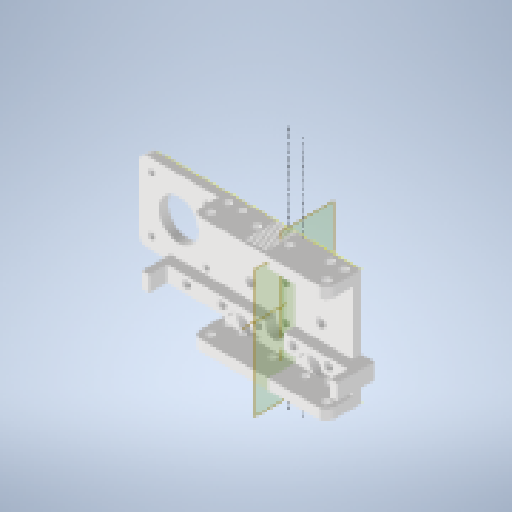
# Autodesk Inventor part: Frontside
Saved by Autodesk Inventor 2023 (Build 270158000, 158)
## iProperties
Created: 2023-08-31
Part Number: Frontside
Material: Generic
Document SubType Name: Modeling
Designer: Felix
Density: 1 g/cm^3
Appearance: Default
Author: Felix
Autodesk Inventor part; units mm, degrees
ref_plane "YZ Plane" through (0, 0, 0) normal (1, 0, 0) x (0, 1, 0)
ref_plane "XZ Plane" through (0, 0, 0) normal (0, 1, 0) x (-1, 0, 0)
ref_plane "XY Plane" through (0, 0, 0) normal (0, 0, 1) x (1, 0, 0)
ref_plane "Work Plane1" through (-29.75, -29.75, 0) normal (-1, 0, 0) x (0, 0, 1)
sketch "Sketch2" plane through (-29.75, -29.75, 0) normal (-1, 0, 0) x (0, 0, 1)
  line L0 (0, 32.5371) -> (-3, 32.5371) construction
  line L1 (0, -32.9629) -> (-3, -32.9629) construction
  line L2 (0, 32.5371) -> (5, 32.5371)
  line L3 (5, 32.5371) -> (5, -32.9629)
  line L4 (5, -32.9629) -> (0, -32.9629)
  line L5 (0, -32.9629) -> (0, 32.5371)
  line L6 (5, 32.5371) -> (20, 32.5371)
  line L7 (20, 32.5371) -> (20, 26.5371)
  line L8 (20, 26.5371) -> (5, 26.5371)
  line L9 (5, 26.5371) -> (5, 32.5371)
  line L10 (5, -32.9629) -> (20, -32.9629)
  line L11 (20, -32.9629) -> (20, -26.9629)
  line L12 (20, -26.9629) -> (5, -26.9629)
  line L13 (5, -26.9629) -> (5, -32.9629)
  point P0 (0, 29.75)
  point P1 (20, 29.5371)
  point P2 (5, 26.5371)
  dimension "d0" = 5
  dimension "d1" = 6
  dimension "d2" = 20
  dimension "d3" = 6
  dimension "d4" = 20
  constraints: 24 end point, 6 parallel, 3 horizontal, 3 perpendicular, 1 midpoint, 1 point on line
  measures "d0" distance of L3.end L4.end
  measures "d1" distance between parallel lines of L6 L8
  measures "d2" distance from line of point (20, 29.537) L5
  measures "d3" distance of L10.end L11.end
  measures "d4" distance between parallel lines of L5 L11
extrude "Extrusion1" add sketch "Sketch2" along normal mid plane 75.5
sketch "Sketch3" plane through (-67.5, -3.2129, 5) normal (0, 0, 1) x (1, 0, 0)
  circle A0 centre (17.6, -46.75) radius 2.5 construction
  circle A1 centre (57.6, -46.75) radius 3.6 construction
  circle A2 centre (17.6, -6.75) radius 2.5 construction
  circle A3 centre (57.6, -6.75) radius 3.6 construction
  point P0 (67.5, 3.2129)
hole "Hole1" at (-49.9, -49.9629, 5) at (-49.9, -9.9629, 5) at (-9.9, -9.9629, 5) at (-9.9, -49.9629, 5) direction (0, 0, -1) diameter 15 end through all
sketch "Sketch4" plane through (-67.5, -3.2129, 5) normal (0, 0, 1) x (1, 0, 0)
  circle A0 centre (57.6, -26.75) radius 3.6 construction
  circle A1 centre (17.9, -26.75) radius 2.55 construction
  point P0 (67.5, 3.2129)
hole "Hole2" at (-49.6, -29.9629, 5) at (-9.9, -29.9629, 5) direction (0, 0, -1) diameter 5.5 end through all clearance for "Countersunk Flat Head Screw DIN EN ISO 2009" size "M5" standard "DIN"
hole "Hole3" at (-29.75, -39.9629, 5) at (-29.75, -19.9629, 5) direction (0, 0, -1) diameter 4.5 end through all clearance for "Slotted Cheese Head Screw DIN 84" size "M4" standard "DIN"
sketch "Sketch6" plane through (-67.5, -3.2129, 5) normal (0, 0, 1) x (1, 0, 0)
  line L0 (0, 6) -> (0, -59.5) construction
  line L1 (75.5, -59.5) -> (75.5, 6) construction
  line L2 (0, -53.5) -> (0, 0) construction
  line L3 (-27.25, -44.5) -> (82.75, -44.5)
  line L4 (82.75, -44.5) -> (82.75, -35.5)
  line L5 (82.75, -35.5) -> (-27.25, -35.5)
  line L6 (-27.25, -35.5) -> (-27.25, -44.5)
  circle A0 centre (17.9, -26.75) radius 2.75 construction
  circle A1 centre (57.6, -26.75) radius 2.75 construction
  circle A2 centre (17.9, -26.75) radius 6.5
  circle A3 centre (57.6, -26.75) radius 6.5
  line L7 (75.5, -53.5) -> (0, -53.5) projected
  arc A4 (20.8692, -53.5) -> (14.3308, -53.5) centre (17.6, -46.75) ccw projected
  arc A5 (60.8692, -53.5) -> (54.3308, -53.5) centre (57.6, -46.75) ccw projected
  line L8 (-27.25, -40) -> (82.75, -40) construction
  line L9 (0, -26.75) -> (75.5, -26.75) construction
  circle A6 centre (37.75, -36.75) radius 2.25 projected
  circle A7 centre (37.75, -36.75) radius 2.25 projected
  circle A8 centre (37.75, -36.75) radius 5.5
  point P0 (67.5, 3.2129)
  point P1 (67.75, -40)
  point P2 (47.75, -40)
  point P3 (27.75, -40)
  point P4 (7.75, -40)
  point P5 (-12.25, -40)
  point P6 (52.8231, -32.1581)
  point P7 (62.2904, -32.25)
  point P8 (52.9096, -32.25)
  point P9 (62.3769, -32.1581)
  point P10 (13.1231, -32.1581)
  point P11 (22.5904, -32.25)
  point P12 (13.2096, -32.25)
  point P13 (22.6769, -32.1581)
  point P14 (37.75, -26.75)
  point P15 (10.4455, -44.5)
  point P16 (24.7545, -44.5)
  point P17 (50.4455, -44.5)
  point P18 (64.7545, -44.5)
  point P19 (43.1061, -35.5)
  point P20 (32.3939, -35.5)
  point P21 (35.8792, -35.5)
  point P22 (39.6208, -35.5)
  dimension "d28" = 20
  dimension "d29" = 20
  dimension "d30" = 20
  dimension "d31" = 20
  dimension "d33" = 9
  dimension "d34" = 110
  dimension "d36" = 15
  dimension "d38" = 13
  dimension "d39" = 13
  dimension "d56" = 15
  dimension "d57" = 9
  dimension "d58" = 10
  dimension "d59" = 11
  constraints: 12 end point, 6 midpoint, 4 point on line, 3 centre point, 3 coincident, 2 horizontal, 2 parallel, 1 perpendicular
  measures "d28" distance of point (-12.25, -40) point (7.75, -40)
  measures "d29" distance of point (7.75, -40) point (27.75, -40)
  measures "d30" distance of point (27.75, -40) point (47.75, -40)
  measures "d31" distance of point (47.75, -40) point (67.75, -40)
  measures "d33" distance between parallel lines of L5 L3
  measures "d34" distance between parallel lines of L6 L4
  measures "d36" distance from line of point (67.75, -40) L4
  measures "d38" diameter of A2
  measures "d39" diameter of A3
  measures "d56" distance from line of L6 point (-12.25, -40)
  measures "d57" distance between parallel lines of L7 L3
  measures "d58" horizontal distance of point (27.75, -40) point (37.75, -26.75)
  measures "d59" diameter of A8
extrude "Extrusion2" add sketch "Sketch6" along normal blind 6 and the other way blind 5 contours L6 L5 A8 L4 L3 A5 A4
sketch "Sketch7" plane through (-67.5, -3.2129, 11) normal (0, 0, 1) x (1, 0, 0)
  point P0 (67.5, 3.2129)
  point P1 (-12.25, -40)
  point P2 (7.75, -40)
  point P3 (27.75, -40)
  point P4 (47.75, -40)
  point P5 (67.75, -40)
hole "Hole4" at (-79.75, -43.2129, 11) at (-59.75, -43.2129, 11) at (-39.75, -43.2129, 11) at (-19.75, -43.2129, 11) at (0.25, -43.2129, 11) direction (0, 0, -1) diameter 4.3 end through all countersink diameter 5 countersink angle 90
sketch "Sketch8" plane through (-67.5, -3.2129, 11) normal (0, 0, 1) x (1, 0, 0)
  line L0 (-27.25, -35.5) -> (-27.25, -44.5) projected
  line L1 (82.75, -44.5) -> (82.75, -35.5) projected
  line L2 (82.75, -35.5) -> (-27.25, -35.5) construction
  line L3 (-27.25, -44.5) -> (82.75, -44.5) construction
  line L4 (-27.25, -35.5) -> (-23.25, -35.5)
  line L5 (-23.25, -35.5) -> (-23.25, -44.5)
  line L6 (-23.25, -44.5) -> (-27.25, -44.5)
  line L7 (-27.25, -44.5) -> (-27.25, -35.5)
  line L8 (82.75, -35.5) -> (-27.25, -35.5) construction
  line L9 (82.75, -44.5) -> (78.75, -44.5)
  line L10 (78.75, -44.5) -> (78.75, -35.5)
  line L11 (78.75, -35.5) -> (82.75, -35.5)
  line L12 (82.75, -35.5) -> (82.75, -44.5)
  point P0 (67.5, 3.2129)
  point P1 (13.2096, -23.25)
  point P2 (13.2096, -32.25)
  point P3 (62.2904, -23.25)
  dimension "d51" = 4
  dimension "d52" = 4
  constraints: 16 end point, 4 parallel, 2 horizontal, 2 perpendicular, 5 other
  measures "d51" distance of L5.end L6.end
  measures "d52" distance of L10.end L11.end
extrude "Extrusion3" add sketch "Sketch8" along normal blind 11
sketch "Sketch9" plane through (8, -62.7129, 0) normal (0, 0, -1) x (-1, 0, 0)
  line L0 (113.5, 58.5) -> (82.5, 58.5) construction
  line L1 (82.5, 58.5) -> (82.5, 27.5) construction
  line L2 (82.5, 27.5) -> (113.5, 27.5) construction
  line L3 (113.5, 27.5) -> (113.5, 58.5) construction
  line L4 (113.5, 58.5) -> (82.5, 27.5) construction
  line L5 (82.5, 58.5) -> (113.5, 27.5) construction
  line L6 (75.5, 65.5) -> (75.5, 24) construction
  line L7 (102.75, 24) -> (75.5, 24) construction
  line L8 (120.5, 20.5) -> (75.5, 20.5)
  line L9 (75.5, 20.5) -> (75.5, 65.5)
  line L10 (75.5, 65.5) -> (120.5, 65.5)
  line L11 (120.5, 65.5) -> (120.5, 20.5)
  line L12 (120.5, 20.5) -> (75.5, 65.5) construction
  line L13 (75.5, 20.5) -> (120.5, 65.5) construction
  circle A0 centre (98, 43) radius 11.25
  point P0 (8, 62.7129)
  dimension "d60" = 31
  dimension "d61" = 31
  dimension "d62" = 45
  dimension "d63" = 45
  dimension "d64" = 22.5
  constraints: 24 end point, 4 midpoint, 4 parallel, 2 horizontal, 2 perpendicular, 1 centre point, 1 coincident
  measures "d60" distance of L2.end L1.end
  measures "d61" distance of L1.end L0.end
  measures "d62" distance of L6.start L10.end
  measures "d63" distance of L6.start L8.end
  measures "d64" diameter of A0
extrude "Extrusion4" add sketch "Sketch9" against normal up to surface (5 mm away)
sketch "Sketch10" plane through (-67.5, -3.2129, 5) normal (0, 0, 1) x (1, 0, 0)
  point P0 (67.5, 3.2129)
  point P1 (-38, -1)
  point P2 (-38, -32)
  point P3 (-7, -32)
  point P4 (-7, -1)
hole "Hole5" at (-105.5, -35.2129, 5) at (-74.5, -35.2129, 5) at (-74.5, -4.2129, 5) at (-105.5, -4.2129, 5) direction (0, 0, -1) diameter 3.6 depth 8 clearance for "Countersunk Flat Head Screw DIN EN ISO 2009" size "M3" standard "DIN"
fillet "Fillet1" radius 5 8 edges at (-67.5, -52.2129, 5) (-67.5, -0.2129, 20) (-67.5, -59.7129, 20) (8, -59.7129, 20) (8, -0.2129, 20) (-94.75, -42.2129, 2.5) (-112.5, -42.2129, 2.5) (-112.5, 2.7871, 2.5)
ref_plane "Work Plane2" through (-24.7, -35.7634, 20.0758) normal (-1, 0, 0) x (0, 0, 1)
sketch "Sketch11" plane through (-24.7, -35.7634, 20.0758) normal (-1, 0, 0) x (0, 0, 1)
  line L0 (-20.0758, -26.9495) -> (-5.0758, -26.9495) construction
  line L1 (-20.0758, -27.1495) -> (-20.0758, -26.9495) construction
  line L2 (-5.0758, -26.9495) -> (-20.0758, -26.9495) construction
  line L3 (-19.0758, -27.1495) -> (-19.0758, -26.9495) construction
  arc A0 (-20.0758, -27.1495) -> (-19.0758, -27.1495) centre (-19.5758, -27.1495) ccw construction
  arc A1 (-18.0758, -27.1495) -> (-17.0758, -27.1495) centre (-17.5758, -27.1495) ccw construction
  line L4 (-18.0758, -27.1495) -> (-18.0758, -26.9495) construction
  line L5 (-17.0758, -27.1495) -> (-17.0758, -26.9495) construction
  arc A2 (-16.0758, -27.1495) -> (-15.0758, -27.1495) centre (-15.5758, -27.1495) ccw construction
  line L6 (-16.0758, -27.1495) -> (-16.0758, -26.9495) construction
  line L7 (-15.0758, -27.1495) -> (-15.0758, -26.9495) construction
  arc A3 (-14.0758, -27.1495) -> (-13.0758, -27.1495) centre (-13.5758, -27.1495) ccw construction
  line L8 (-14.0758, -27.1495) -> (-14.0758, -26.9495) construction
  line L9 (-13.0758, -27.1495) -> (-13.0758, -26.9495) construction
  arc A4 (-12.0758, -27.1495) -> (-11.0758, -27.1495) centre (-11.5758, -27.1495) ccw construction
  line L10 (-12.0758, -27.1495) -> (-12.0758, -26.9495) construction
  line L11 (-11.0758, -27.1495) -> (-11.0758, -26.9495) construction
  arc A5 (-10.0758, -27.1495) -> (-9.0758, -27.1495) centre (-9.5758, -27.1495) ccw construction
  line L12 (-10.0758, -27.1495) -> (-10.0758, -26.9495) construction
  line L13 (-9.0758, -27.1495) -> (-9.0758, -26.9495) construction
  arc A6 (-8.0758, -27.1495) -> (-7.0758, -27.1495) centre (-7.5758, -27.1495) ccw construction
  line L14 (-8.0758, -27.1495) -> (-8.0758, -26.9495) construction
  line L15 (-7.0758, -27.1495) -> (-7.0758, -26.9495) construction
  arc A7 (-6.0758, -27.1495) -> (-5.0758, -27.1495) centre (-5.5758, -27.1495) ccw construction
  line L16 (-6.0758, -27.1495) -> (-6.0758, -26.9495) construction
  line L17 (-5.0758, -27.1495) -> (-5.0758, -26.9495) construction
  arc A8 (-4.0758, -27.1495) -> (-3.0758, -27.1495) centre (-3.5758, -27.1495) ccw construction
  line L18 (-4.0758, -27.1495) -> (-4.0758, -26.9495) construction
  line L19 (-3.0758, -27.1495) -> (-3.0758, -26.9495) construction
  arc A9 (-2.0758, -27.1495) -> (-1.0758, -27.1495) centre (-1.5758, -27.1495) ccw construction
  line L20 (-2.0758, -27.1495) -> (-2.0758, -26.9495) construction
  line L21 (-1.0758, -27.1495) -> (-1.0758, -26.9495) construction
  line L22 (-20.0758, -26.9495) -> (-1.0758, -26.9495) construction
  line L23 (-0.0758, -26.9495) -> (-5.0758, -26.9495) construction
  line L24 (-20.0758, -26.9495) -> (-20.0758, -23.9495) projected
  line L25 (-20.0758, -26.4495) -> (-20.0758, -26.2495) construction
  line L26 (-19.0758, -26.4495) -> (-19.0758, -26.2495)
  line L27 (-18.0758, -26.4495) -> (-18.0758, -26.2495)
  line L28 (-17.0758, -26.4495) -> (-17.0758, -26.2495)
  line L29 (-16.0758, -26.4495) -> (-16.0758, -26.2495)
  line L30 (-15.0758, -26.4495) -> (-15.0758, -26.2495)
  arc A10 (-20.0758, -26.4495) -> (-19.0758, -26.4495) centre (-19.5758, -26.4495) ccw
  arc A11 (-18.0758, -26.4495) -> (-17.0758, -26.4495) centre (-17.5758, -26.4495) ccw
  arc A12 (-16.0758, -26.4495) -> (-15.0758, -26.4495) centre (-15.5758, -26.4495) ccw
  line L31 (-20.0758, -26.2495) -> (-1.0758, -26.2495)
  line L32 (-14.0758, -26.4495) -> (-14.0758, -26.2495)
  arc A13 (-14.0758, -26.4495) -> (-13.0758, -26.4495) centre (-13.5758, -26.4495) ccw
  line L33 (-13.0758, -26.4495) -> (-13.0758, -26.2495)
  line L34 (-12.0758, -26.4495) -> (-12.0758, -26.2495)
  arc A14 (-12.0758, -26.4495) -> (-11.0758, -26.4495) centre (-11.5758, -26.4495) ccw
  line L35 (-11.0758, -26.4495) -> (-11.0758, -26.2495)
  line L36 (-10.0758, -26.4495) -> (-10.0758, -26.2495)
  line L37 (-9.0758, -26.4495) -> (-9.0758, -26.2495)
  arc A15 (-10.0758, -26.4495) -> (-9.0758, -26.4495) centre (-9.5758, -26.4495) ccw
  line L38 (-8.0758, -26.4495) -> (-8.0758, -26.2495)
  arc A16 (-8.0758, -26.4495) -> (-7.0758, -26.4495) centre (-7.5758, -26.4495) ccw
  line L39 (-7.0758, -26.4495) -> (-7.0758, -26.2495)
  line L40 (-6.0758, -26.4495) -> (-6.0758, -26.2495)
  arc A17 (-6.0758, -26.4495) -> (-5.0758, -26.4495) centre (-5.5758, -26.4495) ccw
  line L41 (-5.0758, -26.4495) -> (-5.0758, -26.2495)
  arc A18 (-4.0758, -26.4495) -> (-3.0758, -26.4495) centre (-3.5758, -26.4495) ccw
  line L42 (-4.0758, -26.4495) -> (-4.0758, -26.2495)
  line L43 (-3.0758, -26.4495) -> (-3.0758, -26.2495)
  line L44 (-2.0758, -26.4495) -> (-2.0758, -26.2495)
  line L45 (-1.0758, -26.4495) -> (-1.0758, -26.2495)
  arc A19 (-2.0758, -26.4495) -> (-1.0758, -26.4495) centre (-1.5758, -26.4495) ccw
  line L46 (-1.5758, -26.9495) -> (-19.5758, -26.9495)
  point P0 (-20.0758, 35.7634)
  point P1 (-2.0758, -26.9495)
  point P2 (-3.0758, -26.9495)
  point P3 (-4.0758, -26.9495)
  point P4 (-6.0758, -26.9495)
  point P5 (-7.0758, -26.9495)
  point P6 (-8.0758, -26.9495)
  point P7 (-9.0758, -26.9495)
  point P8 (-10.0758, -26.9495)
  point P9 (-11.0758, -26.9495)
  point P10 (-12.0758, -26.9495)
  point P11 (-13.0758, -26.9495)
  point P12 (-14.0758, -26.9495)
  point P13 (-15.0758, -26.9495)
  point P14 (-17.0758, -26.9495)
  point P15 (-19.0758, -26.9495)
  point P16 (-5.0758, -26.2495)
  point P17 (-0.0758, -26.2495)
  point P18 (-3.5758, -26.9495)
  point P19 (-2.0758, -26.2495)
  point P20 (-3.0758, -26.2495)
  point P21 (-5.5758, -26.9495)
  point P22 (-4.0758, -26.2495)
  point P23 (-5.0758, -26.2495)
  point P24 (-7.5758, -26.9495)
  point P25 (-6.0758, -26.2495)
  point P26 (-7.0758, -26.2495)
  point P27 (-9.5758, -26.9495)
  point P28 (-8.0758, -26.2495)
  point P29 (-9.0758, -26.2495)
  point P30 (-11.5758, -26.9495)
  point P31 (-10.0758, -26.2495)
  point P32 (-11.0758, -26.2495)
  point P33 (-13.5758, -26.9495)
  point P34 (-12.0758, -26.2495)
  point P35 (-13.0758, -26.2495)
  point P36 (-15.5758, -26.9495)
  point P37 (-14.0758, -26.2495)
  point P38 (-15.0758, -26.2495)
  point P39 (-17.5758, -26.9495)
  point P40 (-16.0758, -26.2495)
  point P41 (-17.0758, -26.2495)
  point P42 (-18.0758, -26.2495)
  point P43 (-19.0758, -26.2495)
  dimension "d76" = 0.2
  dimension "d77" = 0.5
  dimension "d80" = 2
  dimension "d135" = 0.7
  constraints: 86 end point, 42 point on circle, 20 centre point, 2 perpendicular, 2 tangent, 1 collinear, 1 horizontal, 1 point on line, 1 vertical, 155 other
  measures "d76" distance from line of L0 A0.centre
  measures "d77" radius of A0
  measures "d80" distance of A0.centre A1.centre
  measures "d135" distance of A0.centre A10.centre
extrude "Extrusion5" cut sketch "Sketch11" along normal mid plane 12 contours A10 L26 L31 L27 A11 L46 | A11 L28 L31 L29 A12 L46 | A12 L30 L31 L32 A13 L46 | A13 L33 L31 L34 A14 L46 | A14 L35 L31 L36 A15 L46 | A15 L37 L31 L38 A16 L46 | A16 L39 L31 L40 A17 L46 | A17 L41 L31 L42 A18 L46 | A18 L43 L31 L44 A19 L46
sketch "Sketch12" plane through (-62.5, -62.7129, 20) normal (0, -1, 0) x (1, 0, 0)
  arc A0 (26.95, -15.5) -> (30.15, -15.5) centre (28.55, -15.5) ccw construction
  line L0 (30.15, -7.5) -> (30.15, -15.5) construction
  arc A1 (30.15, -7.5) -> (26.95, -7.5) centre (28.55, -7.5) ccw construction
  line L1 (26.95, -15.5) -> (26.95, -7.5) construction
  arc A2 (45.45, -15.5) -> (48.65, -15.5) centre (47.05, -15.5) ccw construction
  line L2 (48.65, -7.5) -> (48.65, -15.5) construction
  arc A3 (48.65, -7.5) -> (45.45, -7.5) centre (47.05, -7.5) ccw construction
  line L3 (45.45, -15.5) -> (45.45, -7.5) construction
  line L4 (28.55, -15.5) -> (28.55, -7.5) construction
  line L5 (47.05, -15.5) -> (47.05, -7.5) construction
  point P0 (62.5, -20)
  point P1 (28.55, -11.5)
  point P2 (47.05, -11.5)
  constraints: 4 end point, 2 midpoint, 2 vertical
hole "Hole6" at (-33.95, -62.7129, 8.5) at (-15.45, -62.7129, 8.5) direction (0, 1, 0) diameter 4.3 depth 6 countersink diameter 4.5 countersink angle 90
sketch "Sketch13" plane through (15.25, -38.7129, 0) normal (0, 0, -1) x (-1, 0, 0)
  line L0 (48.95, 90.7616) -> (48.95, -48.3769) construction
  line L1 (39.95, 90.7616) -> (39.95, -48.3769) construction
  line L2 (12.25, -24) -> (77.75, -24) construction
  line L3 (12.25, 41.5) -> (77.75, 41.5) construction
  line L4 (39.95, -24) -> (48.95, 41.5) construction
  line L5 (7.25, 41.5) -> (122.75, 41.5) construction
  line L6 (39.95, 41.5) -> (48.95, -24) construction
  line L7 (7.25, -24) -> (82.75, -24) construction
  point P0 (15.25, 38.7129)
  point P1 (45.95, -24)
  point P2 (44.45, 8.75)
  constraints: 8 end point, 8 point on line, 2 vertical, 1 midpoint, 4 other
pattern_circular "Circular Pattern1" count 2 over 360 about axis through (-29.2, -29.9629, 0) along (0, 0, -1) of "Extrusion5", "Hole6"
sketch "Sketch17" plane through (-62.5, -62.7129, 20) normal (0, -1, 0) x (1, 0, 0)
  circle A0 centre (0, -15) radius 1.7 projected
  circle A1 centre (0, -5) radius 1.7 projected
  circle A2 centre (8, -15) radius 1.7 projected
  circle A3 centre (65.5, -15) radius 1.7 projected
  circle A4 centre (57.5, -15) radius 1.7 projected
  circle A5 centre (65.5, -5) radius 1.7 projected
  point P0 (62.5, -20)
hole "Hole9" at (3, -62.7129, 15) at (3, -62.7129, 5) at (-5, -62.7129, 5) at (-54.5, -62.7129, 5) at (-62.5, -62.7129, 5) at (-62.5, -62.7129, 15) direction (0, 1, 0) diameter 4.3 depth 6 countersink diameter 4.5 countersink angle 90
sketch "Sketch18" plane through (-62.5, 2.7871, 20) normal (0, 1, 0) x (1, 0, 0)
  circle A0 centre (65.5, 5) radius 1.7 projected
  circle A1 centre (65.5, 15) radius 1.7 projected
  circle A2 centre (57.5, 15) radius 1.7 projected
  circle A3 centre (0, 5) radius 1.7 projected
  circle A4 centre (0, 15) radius 1.7 projected
  circle A5 centre (8, 15) radius 1.7 projected
  point P0 (62.5, 20)
hole "Hole10" at (-54.5, 2.7871, 5) at (-62.5, 2.7871, 5) at (-62.5, 2.7871, 15) at (3, 2.7871, 5) at (-5, 2.7871, 5) at (3, 2.7871, 15) direction (0, -1, 0) diameter 4.3 depth 6 countersink diameter 4.5 countersink angle 90
sketch "Sketch19" plane through (-67.5, -3.2129, 22) normal (0, 0, 1) x (1, 0, 0)
  line L0 (-23.25, -44.5) -> (-23.25, -35.5) projected
  line L1 (-23.25, -35.5) -> (-27.25, -35.5) projected
  line L2 (-27.25, -35.5) -> (-27.25, -44.5) projected
  line L3 (-27.25, -44.5) -> (-23.25, -44.5) projected
  line L4 (78.75, -35.5) -> (78.75, -44.5) projected
  line L5 (78.75, -44.5) -> (82.75, -44.5) projected
  line L6 (82.75, -44.5) -> (82.75, -35.5) projected
  line L7 (82.75, -35.5) -> (78.75, -35.5) projected
  point P0 (67.5, 3.2129)
extrude "Extrusion6" cut sketch "Sketch19" against normal blind 1
equation "\"d3\" = d1"
equation "\"d4\" = d2"
equation "\"d29\" = d28"
equation "\"d30\" = d28"
equation "\"d31\" = d28"
equation "\"d39\" = d38"
equation "\"d56\" = d36"
body "Solid1"
